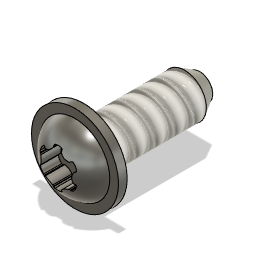
Kunststoff Dome 3er v3 (Autodesk Fusion 360 archive; units mm, degrees)
design "Runde Torxschraube mit Unterlegscheibe, gewindeformend, grobe Ausführung 30° 3x8 C-Stahl Schwarz"
description: Runde Torxschraube mit Unterlegscheibe, gewindeformend, grobe Ausführung 30° 3x8-TR10, C-Stahl, Schwarz
part number: Runde Torxschraube mit Unterlegscheibe, gewindeformend, grobe Ausführung 30° 3x8-TR10, C-Stahl, Schwarz
Autodesk Fusion 360 part; units mm, degrees
sketch "Sketch1" plane through (0, 0, 0) normal (0, 1, 0) x (1, 0, 0)
  line L0 (-1.5, 8) -> (0, 8)
  line L1 (-1.5, 8) -> (-1.5, 0)
  line L2 (-1.5, 0) -> (-3, 0)
  line L3 (-3, 0) -> (-3, -0.6)
  line L4 (0, 8) -> (0, -2.1)
  line L5 (-3, -0.6) -> (-2.4, -0.6)
  arc A0 (-2.4, -0.6) -> (0, -2.1) centre (0, 0.57) ccw
  dimension "d119" = 8
  dimension "d128" = 6
  dimension "d129" = 3
  dimension "d131" = 0.6
  dimension "d132" = 2.1
  constraint perpendicular L1 L2
  constraint perpendicular L2 L3
  constraint perpendicular L0 L4
  constraint vertical L4
  constraint coincident origin L4
  constraint vertical L1
  constraint coincident origin L2
  constraint perpendicular L3 L5
  constraint equal L3 L5
  constraint coincident L4 A0.centre
  constraint coincident L4 A0.end
  measures "d119" distance of L0.start L1.end
  measures "d131" distance of L2.end L3.end
  measures "d132" distance of L2 L4.end
revolve "Revolve1" add sketch "Sketch1" angle 360 about axis through (0, 0, -8) along (0, 0, 1)
ref_plane "WorkPlane2" through (0, 0, 2.1) normal (0, 0, 1) x (1, 0, 0)
sketch "Sketch2" plane through (0, 0, 2.1) normal (0, 0, 1) x (1, 0, 0)
  circle A0 centre (0, 0) radius 1.3298 construction
  line L0 (0, 1.3298) -> (0, -1.3298) construction
  line L1 (1.3298, 0) -> (-1.3298, 0) construction
  arc A1 (-0.8121, 0.8168) -> (-0.3013, 1.1117) centre (-0.9015, 1.5614) ccw
  circle A2 centre (0, 0) radius 1.35
  line L2 (-0.2837, 1.2264) -> (-0.2801, 1.1859)
  line L3 (-0.9015, 1.5614) -> (0, 0) construction
  arc A3 (-0.2305, 1.3096) -> (-0.2837, 1.2264) centre (-0.203, 1.2334) ccw
  circle A4 centre (0, 0) radius 1.053 construction
  arc A5 (-0.3013, 1.1117) -> (-0.2801, 1.1859) centre (-0.3877, 1.1765) ccw
  line L4 (-0.9202, 0.8589) -> (-0.8869, 0.8356)
  arc A6 (-0.8869, 0.8356) -> (-0.8121, 0.8168) centre (-0.825, 0.924) ccw
  arc A7 (-0.9202, 0.8589) -> (-1.0189, 0.8545) centre (-0.9667, 0.7925) ccw
  line L5 (-1.0189, 0.8545) -> (0, 0)
  line L6 (-0.3092, 1.3141) -> (0, 0) construction
  arc A8 (0.2305, 1.3096) -> (-0.2305, 1.3096) centre (0, 0.6718) ccw
  line L7 (0.2305, 1.3096) -> (0, 0)
  point P0 (0.2305, 1.3096)
  point P1 (0, 1.35)
  dimension "d91" = 2.7
  dimension "d92" = 2.6595
  dimension "d98" = 30
  dimension "d100" = 0.081
  dimension "d102" = 2.106
  dimension "d103" = 0.108
  dimension "d104" = 0.0405
  dimension "d109" = 5
  dimension "d110" = 13.239
  constraint coincident A0 L0.start
  constraint coincident A0 L0.end
  constraint vertical L0
  constraint coincident A0.centre L0
  constraint coincident A0 L1.start
  constraint coincident A0 L1.end
  constraint coincident A0.centre L1
  constraint horizontal L1
  constraint concentric A0 A2
  constraint coincident A1.centre L3.start
  constraint tangent L2 A3
  constraint tangent A1 A4
  constraint concentric A0 A4
  constraint tangent A1 A5
  constraint tangent L2 A5
  constraint coincident A0 A3.start
  constraint symmetric L3 L2.start L4.start
  constraint symmetric L3 A3.start A7.end
  constraint symmetric L3 A3 A7
  constraint symmetric L3 L2.end L4.end
  constraint symmetric L3 A1.end A1.start
  constraint symmetric L3 A5 A6
  constraint coincident A1.start A6.end
  constraint coincident A0.centre A2.centre
  constraint coincident A2 L6.start
  constraint tangent A5 L6
  constraint symmetric L0 A3.start P0
  constraint coincident A2 P1
  constraint coincident L0 P1
  constraint coincident P1 A8
  constraint coincident P0 A8.start
  constraint tangent A3 A8
  measures "d91" diameter of A2
  measures "d92" diameter of A0
  measures "d98" angle of L0 L3
  measures "d100" radius of A3
  measures "d102" diameter of A4
  measures "d103" radius of A5
  measures "d104" vertical distance of L2.start L2.end
  measures "d109" angle of L0 L2
  measures "d110" angle of L0 L6
extrude "Extrude5" cut sketch "Sketch2" against normal blind 1.6 contours A1 L2 A3 A5 L4 A6 A7 L5 A8 L7
pattern_circular "C-Pattern1" count 6 over 360 about axis through (0, 0, 1.75) along (0, 0, 1) of "Extrude5"
sketch "Sketch5" plane through (0, 0, 0) normal (0, 1, 0) x (1, 0, 0)
  line L0 (-1.5, 8) -> (0, 8)
  line L1 (-1.5, 6.9608) -> (-0.9, 8)
  line L2 (-1.5, 8) -> (-1.5, 0)
  line L3 (3, 0) -> (-3, 0)
  dimension "d40" = 0.6
  dimension "d126" = 30
  constraint coincident L0 L1.end
  constraint coincident L0.start L2.start
  constraint perpendicular L0 L2
  constraint coincident L1.start L2
  constraint coincident L2.end L3
  measures "d40" distance of L0.start L1.end
  measures "d126" angle of L1 L2
thread "Thread1" "Metric Tapping Threads for Plastics 3.0 3x1.34 h14" major diameter 3 minor diameter 1.66 pitch 1.34 angle 30 resizes the face on face at (-1.4981, 0.0748, -2.6667)
revolve "Revolve2" cut sketch "Sketch5" angle 360 about axis through (0, 0, 1.75) along (0, 0, 1)
equation "NLG = 8 mm"
equation "KOH = 2.1 mm"
equation "KOD = 6 mm"
equation "NND = 3 mm"
equation "SDM = 2.7 mm"
equation "d40 = NND * 0.2"
equation "INTI = 1.6 mm"
equation "d91 = SDM"
equation "d92 = d91 * 0.985"
equation "d100 = SDM * 0.03"
equation "d102 = SDM * 0.78"
equation "d103 = SDM * 0.04"
equation "d104 = SDM * 0.015"
equation "d112 = -INTI"
equation "d119 = NLG"
equation "d125 = KOH"
equation "d128 = KOD"
equation "d129 = NND"
equation "KOF = 0.6 mm"
equation "d131 = KOF"
equation "d132 = KOH"
